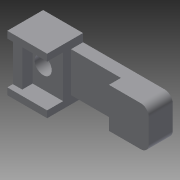
# Autodesk Inventor part: CradleTop
Saved by Autodesk Inventor 2014 SP1 (Build 180222100, 222)
## iProperties
Created: 2017-05-14
Part Number: CradleTop
Material: Generic
Document SubType Name: Modeling
Designer: danielsikar
Density: 1 g/cm^3
Appearance: Default
Author: danielsikar
Autodesk Inventor part; units mm, degrees
ref_plane "YZ Plane" through (0, 0, 0) normal (1, 0, 0) x (0, 1, 0)
ref_plane "XZ Plane" through (0, 0, 0) normal (0, 1, 0) x (-1, 0, 0)
ref_plane "Work Plane1" through (-6, 33, 48.75) normal (0, 1, 0) x (0, 0, 1)
sketch "Sketch1" plane through (-6, 33, 48.75) normal (0, 1, 0) x (0, 0, 1)
  arc A0 (5, 22.5) -> (3, 24.5) centre (3, 22.5) ccw projected
  line L0 (3, 24.5) -> (-3, 24.5) projected
  arc A1 (-3, 24.5) -> (-5, 22.5) centre (-3, 22.5) ccw projected
  line L1 (-5, 22.5) -> (-5, 14.5) projected
  line L2 (5, 14.5) -> (5, 22.5) projected
  line L3 (5, 4.5) -> (5, 14.5) projected
  line L4 (-5, 4.5) -> (-5, 14.5) projected
  line L5 (-5, 14.5) -> (5, 14.5) projected
  line L6 (5, -8) -> (-5, -8) projected
  line L7 (-5, 2) -> (-5, -8) projected
  line L8 (5, 2) -> (5, -8) projected
  line L9 (-5, 4.6724) -> (-5, 1.6802)
  line L10 (5, 1.6802) -> (5, 5.5636)
  point P0 (-48.75, 6)
  constraints: 4 end point, 4 point on line
extrude "Extrusion1" add sketch "Sketch1" against normal blind 3
sketch "Sketch2" plane through (-6, 30, 48.75) normal (0, -1, 0) x (1, 0, 0)
  line L0 (24.5, -3) -> (24.5, 3) projected
  arc A0 (24.5, 3) -> (22.5, 5) centre (22.5, 3) ccw projected
  line L1 (22.5, 5) -> (-8, 5) projected
  line L2 (-8, -5) -> (22.5, -5) projected
  arc A1 (22.5, -5) -> (24.5, -3) centre (22.5, -3) ccw projected
  line L3 (14.5, -5) -> (14.5, 5) projected
  point P0 (6, -48.75)
extrude "Extrusion2" add sketch "Sketch2" along normal blind 1.5
sketch "Sketch3" plane through (-6, 30, 48.75) normal (0, -1, 0) x (1, 0, 0)
  line L0 (-8, 5) -> (-8, -5) projected
  circle A0 centre (-3, 0) radius 2.15 projected
  line L1 (2, 5) -> (-8, 5) projected
  line L2 (2, 5) -> (2, -5) projected
  line L3 (2, -5) -> (-8, -5) projected
  line L4 (-8, 5) -> (-8, -5) projected
  point P0 (6, -48.75)
extrude "Extrusion3" add sketch "Sketch3" along normal blind 2
sketch "Sketch4" plane through (-14, 33, 53.75) normal (0, 0, 1) x (1, 0, 0)
  line L0 (0, 0) -> (10, 0)
  line L1 (10, 0) -> (10, -5)
  line L2 (10, -5) -> (0, -5)
  line L3 (0, -5) -> (0, 0)
  point P0 (14, -33)
  constraints: 8 end point, 2 parallel, 1 horizontal, 1 perpendicular
extrude "Extrusion4" add sketch "Sketch4" along normal blind 2
sketch "Sketch5" plane through (16.5, 33, 43.75) normal (0, 0, -1) x (-1, 0, 0)
  line L0 (30.5, -5) -> (20.5, -5) projected
  line L1 (30.5, 0) -> (30.5, -5) projected
  line L2 (30.5, 0) -> (20.5, 0)
  line L3 (20.5, 0) -> (20.5, -5)
  line L4 (20.5, -5) -> (30.5, -5)
  line L5 (30.5, -5) -> (30.5, 0)
  point P0 (16.5, -33)
  constraints: 8 end point, 2 parallel, 1 horizontal, 1 perpendicular
extrude "Extrusion5" add sketch "Sketch5" along normal blind 2
sketch "Sketch6" plane through (-6, 33, 48.75) normal (0, 1, 0) x (1, 0, 0)
  circle A0 centre (-3, 0) radius 2.15 projected
  point P0 (6, 48.75)
extrude "Extrusion6" cut sketch "Sketch6" against normal up to next
sketch "Sketch7" plane through (-6, 28, 48.75) normal (0, -1, 0) x (1, 0, 0)
  line L0 (-8, -7) -> (-8, 7) projected
  line L1 (2, -7) -> (-8, -7) projected
  line L2 (2, 7) -> (2, -7) projected
  line L3 (-8, 7) -> (2, 7) projected
  line L4 (2, -5) -> (-8, -5) projected
  line L5 (2, 5) -> (-8, 5) projected
  point P0 (6, -48.75)
extrude "Extrusion7" add sketch "Sketch7" along normal blind 4 contours L0 L4 L2 L1 | L0 L3 L2 L5
sketch "Sketch8" plane through (-14, 28, 43.75) normal (0, 0, 1) x (1, 0, 0)
  line L0 (0, 0) -> (10, 0) projected
  line L1 (0, 0) -> (0, -4) projected
  line L2 (10, -4) -> (0, -4) projected
  line L3 (10, 0) -> (10, -4) projected
  point P0 (14, -28)
extrude "Extrusion8" cut sketch "Sketch8" against normal blind 0.3
sketch "Sketch9" plane through (-4, 28, 53.75) normal (0, 0, -1) x (-1, 0, 0)
  line L0 (0, 0) -> (10, 0) projected
  line L1 (0, 0) -> (0, -4) projected
  line L2 (10, -4) -> (0, -4) projected
  line L3 (10, 0) -> (10, -4) projected
  point P0 (-4, -28)
extrude "Extrusion9" cut sketch "Sketch9" against normal blind 0.3
sketch "Sketch10" plane through (-6, 28.5, 48.75) normal (0, -1, 0) x (1, 0, 0)
  line L0 (24.5, -3) -> (24.5, 3) projected
  arc A0 (24.5, 3) -> (22.5, 5) centre (22.5, 3) ccw projected
  line L1 (22.5, 5) -> (14.5, 5) projected
  line L2 (14.5, 5) -> (14.5, -5) projected
  line L3 (14.5, -5) -> (22.5, -5) projected
  arc A1 (22.5, -5) -> (24.5, -3) centre (22.5, -3) ccw projected
  point P0 (6, -48.75)
extrude "Extrusion10" add sketch "Sketch10" along normal blind 1.5
sketch "Sketch11" plane through (-6, 28, 48.75) normal (0, -1, 0) x (1, 0, 0)
  line L0 (-8, -5.3) -> (-8, 5.3) projected
  line L1 (-8, -5.3) -> (2, -5.3) projected
  line L2 (-8, 5.3) -> (-5.652, 5.3)
  line L3 (-5.652, 5.3) -> (-5.652, -5.3)
  line L4 (-5.652, -5.3) -> (-8, -5.3)
  line L5 (-8, -5.3) -> (-8, 5.3)
  point P0 (6, -48.75)
  constraints: 8 end point, 2 parallel, 1 horizontal, 1 perpendicular, 1 point on line
extrude "Extrusion11" add sketch "Sketch11" along normal blind 2.6
body "Solid1"
